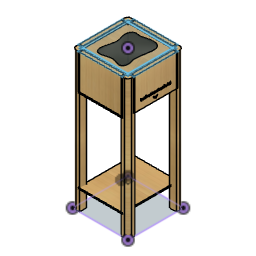
Let-me-fix-it-for-you-Final (Autodesk Fusion 360 design; units mm, degrees)
Autodesk Fusion 360 part; units mm, degrees
(part 1 of 2)
ref_plane "Plan de construction1" through (0, 1000, 0) normal (0, 1, 0) x (0, 0, 1)
sketch "Esquisse1" plane through (0, 1000, 0) normal (0, 1, 0) x (1, 0, 0)
  line L0 (200, 200) -> (-200, 200)
  line L1 (-200, 200) -> (-200, -200)
  line L2 (-200, -200) -> (200, -200)
  line L3 (200, -200) -> (200, 200)
  line L4 (200, 200) -> (-200, -200) construction
  line L5 (-200, 200) -> (200, -200) construction
  dimension "d2" = 400
  constraint horizontal L0
  constraint perpendicular L0 L1
  constraint parallel L0 L2
  constraint parallel L1 L3
  constraint coincident L4 origin
  constraint coincident L5 origin
  constraint equal L0 L1
  measures "d2" distance of L0.start L0.end
sketch "Esquisse2" plane through (0, 0, 0) normal (0, 1, 0) x (1, 0, 0)
  line L0 (200, 200) -> (-200, 200)
  line L1 (-200, 200) -> (-200, -200)
  line L2 (-200, -200) -> (200, -200)
  line L3 (200, -200) -> (200, 200)
  line L4 (-200, 200) -> (-150, 200)
  line L5 (-150, 200) -> (-150, 150)
  line L6 (-150, 150) -> (-200, 150)
  line L7 (-200, 150) -> (-200, 200)
  dimension "d3" = 50
  constraint horizontal L4
  constraint vertical L5
  constraint horizontal L6
  constraint vertical L7
  constraint coincident L0 L1.start
  constraint coincident L1 L6.end
  constraint equal L5 L6
  measures "d3" distance of L5.end L6.end
extrude "Extrusion1" add sketch "Esquisse2" along normal up to surface (1000 mm away) contours L0 L1 L4 L5 L6 L7 makes body 1
fillet "Congé1" radius 25 1 edges at (-200, 500, -200) on bodies 1
pattern_circular "Réseau C1" count 4 over 360 about axis through (0, 1.75, 0) along (0, 1, 0) of bodies 1 makes body 2 at (-150, 333.3333, 166.6667) makes body 3 at (166.6667, 333.3333, 150) makes body 4 at (150, 333.3333, -166.6667)
sketch "Esquisse6" plane through (0, 1000, 0) normal (0, 1, 0) x (1, 0, 0)
  line L0 (200, -160.0001) -> (160.0002, -160.0001)
  line L1 (160.0002, -160.0001) -> (160.0002, 160.0013)
  line L2 (160.0002, 160.0013) -> (200, 160.0013)
  line L3 (200, 160.0013) -> (200, -160.0001)
  line L4 (-160.0013, 200) -> (160.0001, 200)
  line L5 (160.0001, 160.0002) -> (-160.0013, 160.0002)
  line L6 (-160.0013, 160.0002) -> (-160.0013, 200)
  line L7 (160.0001, 200) -> (160.0001, 160.0002)
  line L8 (-200, -160.0013) -> (-200, 160.0001)
  line L9 (-160.0002, 160.0001) -> (-160.0002, -160.0013)
  line L10 (-160.0002, -160.0013) -> (-200, -160.0013)
  line L11 (-200, 160.0001) -> (-160.0002, 160.0001)
  line L12 (160.0013, -200) -> (-160.0001, -200)
  line L13 (-160.0001, -160.0002) -> (160.0013, -160.0002)
  line L14 (160.0013, -160.0002) -> (160.0013, -200)
  line L15 (-160.0001, -200) -> (-160.0001, -160.0002)
  dimension "d15" = 360
  constraint horizontal L0
  constraint vertical L1
  constraint horizontal L2
  constraint vertical L3
extrude "Extrusion2" add sketch "Esquisse6" against normal blind 230 separate body contours L0 L1 L2 L3 makes body 5
extrude "Extrusion3" add sketch "Esquisse6" against normal blind 250 separate body contours L12 L13 L14 L15 | L4 L5 L6 L7 | L8 L9 L10 L11 makes body 6 at (53.3342, 916.6667, 200) makes body 7 at (-160.0009, 916.6667, -53.333) makes body 8 at (53.333, 833.3333, -160.0009)
sketch "Esquisse15" plane through (0, 1000, 0) normal (0, 1, 0) x (1, 0, 0)
  line L0 (-175, 175) -> (175, 175)
  line L1 (175, 175) -> (175, -175)
  line L2 (175, -175) -> (-175, -175)
  line L3 (-175, -175) -> (-175, 175)
  constraint horizontal L0
  constraint vertical L1
  constraint horizontal L2
  constraint vertical L3
ref_plane "Plan de construction8" through (0, 750, 0) normal (0, 1, 0) x (1, 0, 0)
sketch "Esquisse17" plane through (0, 1000, 0) normal (0, 1, 0) x (1, 0, 0)
  line L0 (160, -200) -> (-160, -200)
  line L1 (-160, -200) -> (-160, 200)
  line L2 (-160, 200) -> (160, 200)
  line L3 (160, 200) -> (160, -200)
  constraint horizontal L0
  constraint vertical L1
  constraint horizontal L2
  constraint vertical L3
extrude "Extrusion9" add sketch "Esquisse17" against normal blind 10 from surface at -250 separate body makes body 9
extrude "Extrusion10" cut sketch "Esquisse15" against normal blind 3 bodies 1 2 3 4 5 6 7 8
extrude "Extrusion11" add sketch "Esquisse15" against normal blind 3 separate body makes body 10
ref_plane "Plan de construction9" through (0, 980, 0) normal (0, 1, 0) x (1, 0, 0)
extrude "Extrusion12" cut sketch "Esquisse15" along normal blind 3 from surface at -20 bodies 1 2 3 4 5 6 7 8
extrude "Extrusion13" add sketch "Esquisse15" along normal blind 3 from surface at -20 separate body makes body 11
sketch "Esquisse19" plane through (0, 1000, 0) normal (0, 1, 0) x (1, 0, 0)
  line L0 (107.45, 140.3) -> (-107.45, 140.3)
  line L1 (-107.45, 140.3) -> (-107.45, -140.3)
  line L2 (-107.45, -140.3) -> (107.45, -140.3)
  line L3 (107.45, -140.3) -> (107.45, 140.3)
  line L4 (107.45, 140.3) -> (-107.45, -140.3) construction
  line L5 (-107.45, 140.3) -> (107.45, -140.3) construction
  dimension "d66" = 214.9
  dimension "d67" = 280.6
  constraint horizontal L0
  constraint perpendicular L0 L1
  constraint parallel L0 L2
  constraint parallel L1 L3
  constraint coincident L4 origin
  constraint coincident L5 origin
  measures "d66" distance of L1.end L2.end
  measures "d67" distance of L0.end L1.end
extrude "Extrusion15" add sketch "Esquisse19" along normal blind 6.4 from surface at -17 bodies 11
ref_plane "Plan de construction10" through (0, 997, 0) normal (0, 1, 0) x (1, 0, 0)
extrude "Extrusion17" cut sketch "Esquisse15" against normal blind 3 from surface at -3 bodies 1 2 3 4 5 6 8 11
extrude "Extrusion18" add sketch "Esquisse15" against normal blind 3 from surface at -3 separate body makes body 12
sketch "Esquisse20" plane through (0, 1000, 0) normal (0, 1, 0) x (1, 0, 0)
  spline S0 degree 5 poles (2.9702, -120.1045) (7.0681, -119.8348) (15.2569, -119.7939) (27.4222, -121.4279) (43.0106, -127.0491) (61.2249, -134.4245) (77.5138, -136.2031) (91.0503, -127.6879) (98.8241, -110.0516) (98.8295, -90.0131) (94.6353, -72.3389) (90.1903, -60.1213) (88.8467, -53.3029) (88.4034, -45.7936) (88.4913, -33.5384) (89.8196, -15.0168) (93.0533, 9.1619) (97.7061, 35.6857) (101.4655, 59.537) (103.2857, 79.7063) (102.3989, 96.5235) (98.2065, 110.9745) (90.2444, 123.7985) (77.0958, 133.2881) (58.9031, 137.9279) (37.8289, 138.035) (16.5657, 134.6422) (-2.421, 129.4881) (-17.8557, 124.5172) (-30.8107, 121.6439) (-43.6339, 121.9352) (-58.1106, 124.5676) (-74.1441, 126.1002) (-87.4634, 118.7531) (-96.3647, 103.3877) (-100.3382, 83.9127) (-100.0369, 65.4428) (-96.4821, 49.6829) (-91.3708, 35.4015) (-86.8957, 21.1757) (-84.9832, 5.2069) (-86.8039, -13.7696) (-92.0527, -35.9447) (-98.6926, -60.0391) (-103.9624, -83.9818) (-105.043, -105.3549) (-100.0919, -121.9553) (-88.5831, -132.2499) (-73.2953, -136.0188) (-55.9982, -134.3536) (-37.333, -129.1226) (-21.5591, -124.2663) (-9.3306, -121.4124) (-1.1277, -120.3743) (2.9702, -120.1045) knots 0 0 0 0 0 0 0.02 0.04 0.06 0.08 0.1 0.12 0.14 0.16 0.18 0.2 0.22 0.24 0.26 0.28 0.3 0.32 0.34 0.36 0.38 0.4 0.42 0.44 0.46 0.48 0.5 0.52 0.54 0.56 0.58 0.6 0.62 0.64 0.66 0.68 0.7 0.72 0.74 0.76 0.78 0.8 0.82 0.84 0.86 0.88 0.9 0.92 0.94 0.96 0.98 1 1 1 1 1 1
  line L0 (-41.6235, -123.0399) -> (47.5639, -117.1691)
  line L1 (85.8055, -37.2443) -> (103.3819, 71.9806)
  line L2 (93.3383, -74.908) -> (85.8055, -37.2443)
  line L3 (71.5377, -150.9467) -> (110.117, -96.7951)
  line L4 (108.4038, 100.8562) -> (72.0487, 142.3216)
  line L5 (-102.9243, 107.4984) -> (-95.8249, 27.6746)
  line L6 (-30.9544, 124.4197) -> (-100, 125)
  line L7 (-111.5032, -112.7754) -> (-71.7545, -143.3305)
  point P0 (90.8274, -123.8709)
  point P1 (89.5719, -56.0761)
  point P2 (94.5937, 17.3682)
  point P3 (90.2262, 121.5889)
  point P4 (-5.2152, 128.4762)
  point P5 (-65.4772, 124.7099)
  point P6 (-99.3746, 67.5865)
  point P7 (-86.82, -8.9964)
  point P8 (-91.6288, -128.0529)
  constraint midpoint S0.start L0
  constraint midpoint P2 L1
  constraint midpoint P1 L2
  constraint coincident L1.start L2.end
  constraint midpoint P0 L3
  constraint midpoint P3 L4
  constraint midpoint P6 L5
  constraint midpoint P5 L6
  constraint midpoint P8 L7
extrude "Extrusion19" cut sketch "Esquisse20" against normal blind 3 from surface at -3 bodies 12
sketch "Esquisse29" plane through (200, 0, 0) normal (1, 0, 0) x (0, 0, -1)
  line L0 (-104.418, 836.9255) -> (-104.418, 820.5796)
  line L1 (-104.418, 820.5796) -> (-108.4, 820.5796)
  line L2 (-108.4, 820.5796) -> (-108.4, 836.9255)
  line L3 (-108.4, 836.9255) -> (-104.418, 836.9255)
  spline S0 degree 3 poles (-90.7629, 832.2345) (-89.8554, 831.2476) (-89.4003, 829.8956) (-89.4003, 828.1705) knots 0 0 0 0 1 1 1 1
  line L4 (-89.4003, 828.1705) -> (-89.4003, 820.5796)
  line L5 (-89.4003, 820.5796) -> (-93.3584, 820.5796)
  line L6 (-93.3584, 820.5796) -> (-93.3584, 827.6334)
  spline S1 degree 3 poles (-93.3584, 827.6334) (-93.3584, 828.5039) (-93.5833, 829.1785) (-94.0331, 829.6601) knots 0 0 0 0 1 1 1 1
  spline S2 degree 3 poles (-94.0331, 829.6601) (-94.4829, 830.1416) (-95.0888, 830.3824) (-95.8482, 830.3824) knots 0 0 0 0 1 1 1 1
  spline S3 degree 3 poles (-95.8482, 830.3824) (-96.6075, 830.3824) (-97.2134, 830.1416) (-97.6632, 829.6601) knots 0 0 0 0 1 1 1 1
  spline S4 degree 3 poles (-97.6632, 829.6601) (-98.113, 829.1785) (-98.3379, 828.5039) (-98.3379, 827.6334) knots 0 0 0 0 1 1 1 1
  line L7 (-98.3379, 827.6334) -> (-98.3379, 820.5796)
  line L8 (-98.3379, 820.5796) -> (-102.3199, 820.5796)
  line L9 (-102.3199, 820.5796) -> (-102.3199, 833.5733)
  line L10 (-102.3199, 833.5733) -> (-98.3379, 833.5733)
  line L11 (-98.3379, 833.5733) -> (-98.3379, 831.8508)
  spline S5 degree 3 poles (-98.3379, 831.8508) (-97.9357, 832.425) (-97.3907, 832.8801) (-96.7081, 833.2134) knots 0 0 0 0 1 1 1 1
  spline S6 degree 3 poles (-96.7081, 833.2134) (-96.0254, 833.5468) (-95.2581, 833.7135) (-94.4035, 833.7135) knots 0 0 0 0 1 1 1 1
  spline S7 degree 3 poles (-94.4035, 833.7135) (-92.8822, 833.7135) (-91.6677, 833.2214) (-90.7602, 832.2345) knots 0 0 0 0 1 1 1 1
  line L12 (-90.7602, 832.2345) -> (-90.7629, 832.2345)
  spline S8 degree 3 poles (-85.1643, 820.9765) (-86.048, 821.3654) (-86.7465, 821.8972) (-87.2598, 822.5719) knots 0 0 0 0 1 1 1 1
  spline S9 degree 3 poles (-87.2598, 822.5719) (-87.7731, 823.2466) (-88.0588, 824.0033) (-88.1223, 824.842) knots 0 0 0 0 1 1 1 1
  line L13 (-88.1223, 824.842) -> (-84.188, 824.842)
  spline S10 degree 3 poles (-84.188, 824.842) (-84.1404, 824.3922) (-83.9313, 824.0271) (-83.5583, 823.7466) knots 0 0 0 0 1 1 1 1
  spline S11 degree 3 poles (-83.5583, 823.7466) (-83.1852, 823.4662) (-82.7275, 823.3286) (-82.1851, 823.3286) knots 0 0 0 0 1 1 1 1
  spline S12 degree 3 poles (-82.1851, 823.3286) (-81.6877, 823.3286) (-81.304, 823.4265) (-81.0315, 823.6196) knots 0 0 0 0 1 1 1 1
  spline S13 degree 3 poles (-81.0315, 823.6196) (-80.759, 823.8128) (-80.624, 824.0668) (-80.624, 824.3764) knots 0 0 0 0 1 1 1 1
  spline S14 degree 3 poles (-80.624, 824.3764) (-80.624, 824.7494) (-80.8172, 825.0246) (-81.2061, 825.2019) knots 0 0 0 0 1 1 1 1
  spline S15 degree 3 poles (-81.2061, 825.2019) (-81.5951, 825.3791) (-82.2221, 825.5776) (-83.0926, 825.7945) knots 0 0 0 0 1 1 1 1
  spline S16 degree 3 poles (-83.0926, 825.7945) (-84.0239, 826.0115) (-84.7992, 826.2417) (-85.4209, 826.4824) knots 0 0 0 0 1 1 1 1
  spline S17 degree 3 poles (-85.4209, 826.4824) (-86.0427, 826.7232) (-86.5772, 827.1042) (-87.027, 827.6228) knots 0 0 0 0 1 1 1 1
  spline S18 degree 3 poles (-87.027, 827.6228) (-87.4767, 828.1414) (-87.7016, 828.8452) (-87.7016, 829.7289) knots 0 0 0 0 1 1 1 1
  spline S19 degree 3 poles (-87.7016, 829.7289) (-87.7016, 830.475) (-87.4953, 831.1523) (-87.0852, 831.7662) knots 0 0 0 0 1 1 1 1
  spline S20 degree 3 poles (-87.0852, 831.7662) (-86.6751, 832.38) (-86.0692, 832.8642) (-85.2701, 833.2214) knots 0 0 0 0 1 1 1 1
  spline S21 degree 3 poles (-85.2701, 833.2214) (-84.4711, 833.5786) (-83.5212, 833.7558) (-82.4179, 833.7558) knots 0 0 0 0 1 1 1 1
  spline S22 degree 3 poles (-82.4179, 833.7558) (-80.7881, 833.7558) (-79.5049, 833.351) (-78.5656, 832.544) knots 0 0 0 0 1 1 1 1
  spline S23 degree 3 poles (-78.5656, 832.544) (-77.6263, 831.7371) (-77.0866, 830.6655) (-76.9463, 829.332) knots 0 0 0 0 1 1 1 1
  line L14 (-76.9463, 829.332) -> (-80.624, 829.332)
  spline S24 degree 3 poles (-80.624, 829.332) (-80.6849, 829.7818) (-80.8833, 830.139) (-81.2167, 830.4036) knots 0 0 0 0 1 1 1 1
  spline S25 degree 3 poles (-81.2167, 830.4036) (-81.5501, 830.6681) (-81.9893, 830.8004) (-82.5317, 830.8004) knots 0 0 0 0 1 1 1 1
  spline S26 degree 3 poles (-82.5317, 830.8004) (-82.9974, 830.8004) (-83.3545, 830.7105) (-83.6032, 830.5332) knots 0 0 0 0 1 1 1 1
  spline S27 degree 3 poles (-83.6032, 830.5332) (-83.852, 830.3559) (-83.9763, 830.1099) (-83.9763, 829.8003) knots 0 0 0 0 1 1 1 1
  spline S28 degree 3 poles (-83.9763, 829.8003) (-83.9763, 829.4272) (-83.7779, 829.1494) (-83.3836, 828.9616) knots 0 0 0 0 1 1 1 1
  spline S29 degree 3 poles (-83.3836, 828.9616) (-82.9868, 828.7764) (-82.3703, 828.5885) (-81.5316, 828.4033) knots 0 0 0 0 1 1 1 1
  spline S30 degree 3 poles (-81.5316, 828.4033) (-80.5685, 828.1546) (-79.7853, 827.9112) (-79.1794, 827.6704) knots 0 0 0 0 1 1 1 1
  spline S31 degree 3 poles (-79.1794, 827.6704) (-78.5735, 827.4296) (-78.0417, 827.0407) (-77.584, 826.5062) knots 0 0 0 0 1 1 1 1
  spline S32 degree 3 poles (-77.584, 826.5062) (-77.1263, 825.9718) (-76.8908, 825.2521) (-76.8749, 824.3525) knots 0 0 0 0 1 1 1 1
  spline S33 degree 3 poles (-76.8749, 824.3525) (-76.8749, 823.5905) (-77.0892, 822.9132) (-77.5152, 822.3152) knots 0 0 0 0 1 1 1 1
  spline S34 degree 3 poles (-77.5152, 822.3152) (-77.9412, 821.7173) (-78.555, 821.249) (-79.354, 820.9077) knots 0 0 0 0 1 1 1 1
  spline S35 degree 3 poles (-79.354, 820.9077) (-80.1531, 820.5664) (-81.0818, 820.3944) (-82.1375, 820.3944) knots 0 0 0 0 1 1 1 1
  spline S36 degree 3 poles (-82.1375, 820.3944) (-83.2699, 820.3944) (-84.2806, 820.5875) (-85.1643, 820.9765) knots 0 0 0 0 1 1 1 1
  line L15 (-63.0451, 826.1226) -> (-72.0568, 826.1226)
  spline S37 degree 3 poles (-72.0568, 826.1226) (-71.996, 825.3156) (-71.734, 824.6991) (-71.2763, 824.2705) knots 0 0 0 0 1 1 1 1
  spline S38 degree 3 poles (-71.2763, 824.2705) (-70.8186, 823.8445) (-70.255, 823.6302) (-69.5883, 823.6302) knots 0 0 0 0 1 1 1 1
  spline S39 degree 3 poles (-69.5883, 823.6302) (-68.5961, 823.6302) (-67.9055, 824.0483) (-67.5166, 824.887) knots 0 0 0 0 1 1 1 1
  line L16 (-67.5166, 824.887) -> (-63.278, 824.887)
  spline S40 degree 3 poles (-63.278, 824.887) (-63.4949, 824.0324) (-63.8865, 823.2651) (-64.4527, 822.5825) knots 0 0 0 0 1 1 1 1
  spline S41 degree 3 poles (-64.4527, 822.5825) (-65.0189, 821.8999) (-65.7306, 821.3627) (-66.5826, 820.9765) knots 0 0 0 0 1 1 1 1
  spline S42 degree 3 poles (-66.5826, 820.9765) (-67.4372, 820.5875) (-68.3897, 820.3944) (-69.4454, 820.3944) knots 0 0 0 0 1 1 1 1
  spline S43 degree 3 poles (-69.4454, 820.3944) (-70.718, 820.3944) (-71.8505, 820.6669) (-72.8453, 821.2093) knots 0 0 0 0 1 1 1 1
  spline S44 degree 3 poles (-72.8453, 821.2093) (-73.8401, 821.7517) (-74.6154, 822.5296) (-75.1736, 823.5376) knots 0 0 0 0 1 1 1 1
  spline S45 degree 3 poles (-75.1736, 823.5376) (-75.7319, 824.5457) (-76.0124, 825.7257) (-76.0124, 827.0778) knots 0 0 0 0 1 1 1 1
  spline S46 degree 3 poles (-76.0124, 827.0778) (-76.0124, 828.4298) (-75.7372, 829.6072) (-75.1869, 830.6179) knots 0 0 0 0 1 1 1 1
  spline S47 degree 3 poles (-75.1869, 830.6179) (-74.6365, 831.6259) (-73.8639, 832.4038) (-72.8691, 832.9462) knots 0 0 0 0 1 1 1 1
  spline S48 degree 3 poles (-72.8691, 832.9462) (-71.8769, 833.4886) (-70.7339, 833.7611) (-69.4454, 833.7611) knots 0 0 0 0 1 1 1 1
  spline S49 degree 3 poles (-69.4454, 833.7611) (-68.1569, 833.7611) (-67.0694, 833.4965) (-66.0931, 832.97) knots 0 0 0 0 1 1 1 1
  spline S50 degree 3 poles (-66.0931, 832.97) (-65.1142, 832.4409) (-64.3522, 831.6894) (-63.7992, 830.7105) knots 0 0 0 0 1 1 1 1
  spline S51 degree 3 poles (-63.7992, 830.7105) (-63.2489, 829.7315) (-62.9737, 828.5912) (-62.9737, 827.2868) knots 0 0 0 0 1 1 1 1
  spline S52 degree 3 poles (-62.9737, 827.2868) (-62.9737, 826.9137) (-62.9975, 826.5248) (-63.0425, 826.1226) knots 0 0 0 0 1 1 1 1
  line L17 (-63.0425, 826.1226) -> (-63.0451, 826.1226)
  line L18 (-66.7705, 837.2986) -> (-66.7705, 834.5522)
  line L19 (-66.7705, 834.5522) -> (-72.3823, 836.9044)
  line L20 (-72.3823, 836.9044) -> (-72.3823, 840)
  line L21 (-72.3823, 840) -> (-66.7705, 837.2986)
  spline S53 degree 3 poles (-67.0483, 828.3345) (-67.0483, 829.0171) (-67.2811, 829.5595) (-67.7468, 829.9644) knots 0 0 0 0 1 1 1 1
  spline S54 degree 3 poles (-67.7468, 829.9644) (-68.2124, 830.3692) (-68.7945, 830.5703) (-69.493, 830.5703) knots 0 0 0 0 1 1 1 1
  spline S55 degree 3 poles (-69.493, 830.5703) (-70.1915, 830.5703) (-70.7233, 830.3771) (-71.1811, 829.9882) knots 0 0 0 0 1 1 1 1
  spline S56 degree 3 poles (-71.1811, 829.9882) (-71.6388, 829.5992) (-71.9219, 829.0489) (-72.0304, 828.3345) knots 0 0 0 0 1 1 1 1
  line L22 (-72.0304, 828.3345) -> (-67.0483, 828.3345)
  spline S57 degree 3 poles (-55.9437, 833.097) (-55.2452, 833.5071) (-54.47, 833.7135) (-53.6154, 833.7135) knots 0 0 0 0 1 1 1 1
  line L23 (-53.6154, 833.7135) -> (-53.6154, 829.4987)
  line L24 (-53.6154, 829.4987) -> (-54.7108, 829.4987)
  spline S58 degree 3 poles (-54.7108, 829.4987) (-55.7056, 829.4987) (-56.4491, 829.2844) (-56.9465, 828.8584) knots 0 0 0 0 1 1 1 1
  spline S59 degree 3 poles (-56.9465, 828.8584) (-57.4439, 828.4324) (-57.6926, 827.6836) (-57.6926, 826.6121) knots 0 0 0 0 1 1 1 1
  line L25 (-57.6926, 826.6121) -> (-57.6926, 820.5822)
  line L26 (-57.6926, 820.5822) -> (-61.6746, 820.5822)
  line L27 (-61.6746, 820.5822) -> (-61.6746, 833.5733)
  line L28 (-61.6746, 833.5733) -> (-57.6926, 833.5733)
  line L29 (-57.6926, 833.5733) -> (-57.6926, 831.409)
  spline S60 degree 3 poles (-57.6926, 831.409) (-57.2269, 832.1234) (-56.6449, 832.6869) (-55.9464, 833.097) knots 0 0 0 0 1 1 1 1
  line L30 (-55.9464, 833.097) -> (-55.9437, 833.097)
  line L31 (-40.3201, 826.1226) -> (-49.3318, 826.1226)
  spline S61 degree 3 poles (-49.3318, 826.1226) (-49.2709, 825.3156) (-49.009, 824.6991) (-48.5513, 824.2705) knots 0 0 0 0 1 1 1 1
  spline S62 degree 3 poles (-48.5513, 824.2705) (-48.0935, 823.8445) (-47.53, 823.6302) (-46.8632, 823.6302) knots 0 0 0 0 1 1 1 1
  spline S63 degree 3 poles (-46.8632, 823.6302) (-45.871, 823.6302) (-45.1805, 824.0483) (-44.7915, 824.887) knots 0 0 0 0 1 1 1 1
  line L32 (-44.7915, 824.887) -> (-40.5529, 824.887)
  spline S64 degree 3 poles (-40.5529, 824.887) (-40.7699, 824.0324) (-41.1614, 823.2651) (-41.7276, 822.5825) knots 0 0 0 0 1 1 1 1
  spline S65 degree 3 poles (-41.7276, 822.5825) (-42.2939, 821.8999) (-43.0056, 821.3627) (-43.8575, 820.9765) knots 0 0 0 0 1 1 1 1
  spline S66 degree 3 poles (-43.8575, 820.9765) (-44.7121, 820.5875) (-45.6646, 820.3944) (-46.7203, 820.3944) knots 0 0 0 0 1 1 1 1
  spline S67 degree 3 poles (-46.7203, 820.3944) (-47.993, 820.3944) (-49.1254, 820.6669) (-50.1202, 821.2093) knots 0 0 0 0 1 1 1 1
  spline S68 degree 3 poles (-50.1202, 821.2093) (-51.1151, 821.7517) (-51.8903, 822.5296) (-52.4486, 823.5376) knots 0 0 0 0 1 1 1 1
  spline S69 degree 3 poles (-52.4486, 823.5376) (-53.0068, 824.5457) (-53.2873, 825.7257) (-53.2873, 827.0778) knots 0 0 0 0 1 1 1 1
  spline S70 degree 3 poles (-53.2873, 827.0778) (-53.2873, 828.4298) (-53.0121, 829.6072) (-52.4618, 830.6179) knots 0 0 0 0 1 1 1 1
  spline S71 degree 3 poles (-52.4618, 830.6179) (-51.9115, 831.6259) (-51.1389, 832.4038) (-50.144, 832.9462) knots 0 0 0 0 1 1 1 1
  spline S72 degree 3 poles (-50.144, 832.9462) (-49.1519, 833.4886) (-48.0089, 833.7611) (-46.7203, 833.7611) knots 0 0 0 0 1 1 1 1
  spline S73 degree 3 poles (-46.7203, 833.7611) (-45.4318, 833.7611) (-44.3444, 833.4965) (-43.3681, 832.97) knots 0 0 0 0 1 1 1 1
  spline S74 degree 3 poles (-43.3681, 832.97) (-42.3891, 832.4409) (-41.6271, 831.6894) (-41.0741, 830.7105) knots 0 0 0 0 1 1 1 1
  spline S75 degree 3 poles (-41.0741, 830.7105) (-40.5238, 829.7315) (-40.2486, 828.5912) (-40.2486, 827.2868) knots 0 0 0 0 1 1 1 1
  spline S76 degree 3 poles (-40.2486, 827.2868) (-40.2486, 826.9137) (-40.2724, 826.5248) (-40.3174, 826.1226) knots 0 0 0 0 1 1 1 1
  line L33 (-40.3174, 826.1226) -> (-40.3201, 826.1226)
  spline S77 degree 3 poles (-44.3232, 828.3345) (-44.3232, 829.0171) (-44.556, 829.5595) (-45.0217, 829.9644) knots 0 0 0 0 1 1 1 1
  spline S78 degree 3 poles (-45.0217, 829.9644) (-45.4874, 830.3692) (-46.0695, 830.5703) (-46.768, 830.5703) knots 0 0 0 0 1 1 1 1
  spline S79 degree 3 poles (-46.768, 830.5703) (-47.4665, 830.5703) (-47.9983, 830.3771) (-48.456, 829.9882) knots 0 0 0 0 1 1 1 1
  spline S80 degree 3 poles (-48.456, 829.9882) (-48.9137, 829.5992) (-49.1968, 829.0489) (-49.3053, 828.3345) knots 0 0 0 0 1 1 1 1
  line L34 (-49.3053, 828.3345) -> (-44.3232, 828.3345)
  line L35 (-27.5619, 823.9583) -> (-27.5619, 820.5822)
  line L36 (-27.5619, 820.5822) -> (-29.5886, 820.5822)
  spline S81 degree 3 poles (-29.5886, 820.5822) (-31.0332, 820.5822) (-32.1577, 820.9341) (-32.9646, 821.6406) knots 0 0 0 0 1 1 1 1
  spline S82 degree 3 poles (-32.9646, 821.6406) (-33.7716, 822.347) (-34.1764, 823.5006) (-34.1764, 825.0987) knots 0 0 0 0 1 1 1 1
  line L37 (-34.1764, 825.0987) -> (-34.1764, 830.2686)
  line L38 (-34.1764, 830.2686) -> (-35.7586, 830.2686)
  line L39 (-35.7586, 830.2686) -> (-35.7586, 833.5759)
  line L40 (-35.7586, 833.5759) -> (-34.1764, 833.5759)
  line L41 (-34.1764, 833.5759) -> (-34.1764, 836.743)
  line L42 (-34.1764, 836.743) -> (-30.1945, 836.743)
  line L43 (-30.1945, 836.743) -> (-30.1945, 833.5759)
  line L44 (-30.1945, 833.5759) -> (-27.5857, 833.5759)
  line L45 (-27.5857, 833.5759) -> (-27.5857, 830.2686)
  line L46 (-27.5857, 830.2686) -> (-30.1945, 830.2686)
  line L47 (-30.1945, 830.2686) -> (-30.1945, 825.0537)
  spline S83 degree 3 poles (-30.1945, 825.0537) (-30.1945, 824.6648) (-30.1019, 824.3869) (-29.914, 824.215) knots 0 0 0 0 1 1 1 1
  spline S84 degree 3 poles (-29.914, 824.215) (-29.7288, 824.043) (-29.4166, 823.9583) (-28.9827, 823.9583) knots 0 0 0 0 1 1 1 1
  line L48 (-28.9827, 823.9583) -> (-27.5619, 823.9583)
  spline S85 degree 3 poles (-23.6619, 821.2093) (-24.6779, 821.7517) (-25.4769, 822.5296) (-26.059, 823.5376) knots 0 0 0 0 1 1 1 1
  spline S86 degree 3 poles (-26.059, 823.5376) (-26.6411, 824.5457) (-26.9321, 825.7257) (-26.9321, 827.0778) knots 0 0 0 0 1 1 1 1
  spline S87 degree 3 poles (-26.9321, 827.0778) (-26.9321, 828.4298) (-26.6385, 829.5886) (-26.0484, 830.6046) knots 0 0 0 0 1 1 1 1
  spline S88 degree 3 poles (-26.0484, 830.6046) (-25.4584, 831.6206) (-24.6514, 832.4012) (-23.6275, 832.9436) knots 0 0 0 0 1 1 1 1
  spline S89 degree 3 poles (-23.6275, 832.9436) (-22.6036, 833.486) (-21.4553, 833.7585) (-20.1826, 833.7585) knots 0 0 0 0 1 1 1 1
  spline S90 degree 3 poles (-20.1826, 833.7585) (-18.91, 833.7585) (-17.7617, 833.486) (-16.7378, 832.9436) knots 0 0 0 0 1 1 1 1
  spline S91 degree 3 poles (-16.7378, 832.9436) (-15.7138, 832.4012) (-14.9068, 831.6206) (-14.3168, 830.6046) knots 0 0 0 0 1 1 1 1
  spline S92 degree 3 poles (-14.3168, 830.6046) (-13.7268, 829.5886) (-13.4331, 828.4113) (-13.4331, 827.0778) knots 0 0 0 0 1 1 1 1
  spline S93 degree 3 poles (-13.4331, 827.0778) (-13.4331, 825.7443) (-13.7321, 824.5669) (-14.3301, 823.5509) knots 0 0 0 0 1 1 1 1
  spline S94 degree 3 poles (-14.3301, 823.5509) (-14.928, 822.5349) (-15.7429, 821.7543) (-16.7748, 821.2119) knots 0 0 0 0 1 1 1 1
  spline S95 degree 3 poles (-16.7748, 821.2119) (-17.8067, 820.6695) (-18.9603, 820.397) (-20.2329, 820.397) knots 0 0 0 0 1 1 1 1
  spline S96 degree 3 poles (-20.2329, 820.397) (-21.5056, 820.397) (-22.6512, 820.6695) (-23.6672, 821.2119) knots 0 0 0 0 1 1 1 1
  line L49 (-23.6672, 821.2119) -> (-23.6619, 821.2093)
  spline S97 degree 3 poles (-18.2829, 824.6806) (-17.7485, 825.2389) (-17.4786, 826.0379) (-17.4786, 827.0777) knots 0 0 0 0 1 1 1 1
  spline S98 degree 3 poles (-17.4786, 827.0777) (-17.4786, 828.1176) (-17.7379, 828.9166) (-18.2591, 829.4749) knots 0 0 0 0 1 1 1 1
  spline S99 degree 3 poles (-18.2591, 829.4749) (-18.7803, 830.0331) (-19.4206, 830.3136) (-20.18, 830.3136) knots 0 0 0 0 1 1 1 1
  spline S100 degree 3 poles (-20.18, 830.3136) (-20.9393, 830.3136) (-21.6008, 830.0384) (-22.1114, 829.4881) knots 0 0 0 0 1 1 1 1
  spline S101 degree 3 poles (-22.1114, 829.4881) (-22.6247, 828.9378) (-22.8787, 828.1334) (-22.8787, 827.0777) knots 0 0 0 0 1 1 1 1
  spline S102 degree 3 poles (-22.8787, 827.0777) (-22.8787, 826.0221) (-22.6274, 825.2389) (-22.122, 824.6806) knots 0 0 0 0 1 1 1 1
  spline S103 degree 3 poles (-22.122, 824.6806) (-21.6167, 824.1224) (-20.9843, 823.8419) (-20.225, 823.8419) knots 0 0 0 0 1 1 1 1
  spline S104 degree 3 poles (-20.225, 823.8419) (-19.4656, 823.8419) (-18.8174, 824.1224) (-18.2803, 824.6806) knots 0 0 0 0 1 1 1 1
  line L50 (-18.2803, 824.6806) -> (-18.2829, 824.6806)
  spline S105 degree 3 poles (-0.54, 832.2345) (0.3676, 831.2476) (0.8226, 829.8956) (0.8226, 828.1705) knots 0 0 0 0 1 1 1 1
  line L51 (0.8226, 828.1705) -> (0.8226, 820.5796)
  line L52 (0.8226, 820.5796) -> (-3.1355, 820.5796)
  line L53 (-3.1355, 820.5796) -> (-3.1355, 827.6334)
  spline S106 degree 3 poles (-3.1355, 827.6334) (-3.1355, 828.5039) (-3.3604, 829.1785) (-3.8102, 829.6601) knots 0 0 0 0 1 1 1 1
  spline S107 degree 3 poles (-3.8102, 829.6601) (-4.26, 830.1416) (-4.8659, 830.3824) (-5.6252, 830.3824) knots 0 0 0 0 1 1 1 1
  spline S108 degree 3 poles (-5.6252, 830.3824) (-6.3846, 830.3824) (-6.9905, 830.1416) (-7.4403, 829.6601) knots 0 0 0 0 1 1 1 1
  spline S109 degree 3 poles (-7.4403, 829.6601) (-7.8901, 829.1785) (-8.115, 828.5039) (-8.115, 827.6334) knots 0 0 0 0 1 1 1 1
  line L54 (-8.115, 827.6334) -> (-8.115, 820.5796)
  line L55 (-8.115, 820.5796) -> (-12.0969, 820.5796)
  line L56 (-12.0969, 820.5796) -> (-12.0969, 833.5733)
  line L57 (-12.0969, 833.5733) -> (-8.115, 833.5733)
  line L58 (-8.115, 833.5733) -> (-8.115, 831.8508)
  spline S110 degree 3 poles (-8.115, 831.8508) (-7.7128, 832.425) (-7.1678, 832.8801) (-6.4851, 833.2134) knots 0 0 0 0 1 1 1 1
  spline S111 degree 3 poles (-6.4851, 833.2134) (-5.8025, 833.5468) (-5.0352, 833.7135) (-4.1806, 833.7135) knots 0 0 0 0 1 1 1 1
  spline S112 degree 3 poles (-4.1806, 833.7135) (-2.6593, 833.7135) (-1.4448, 833.2214) (-0.5373, 832.2345) knots 0 0 0 0 1 1 1 1
  line L59 (-0.5373, 832.2345) -> (-0.54, 832.2345)
  spline S113 degree 3 poles (6.9081, 830.6179) (7.4134, 831.6259) (8.0987, 832.4038) (8.9692, 832.9462) knots 0 0 0 0 1 1 1 1
  spline S114 degree 3 poles (8.9692, 832.9462) (9.837, 833.4886) (10.808, 833.7611) (11.8796, 833.7611) knots 0 0 0 0 1 1 1 1
  spline S115 degree 3 poles (11.8796, 833.7611) (12.7342, 833.7611) (13.5121, 833.5812) (14.2185, 833.2267) knots 0 0 0 0 1 1 1 1
  spline S116 degree 3 poles (14.2185, 833.2267) (14.9249, 832.8695) (15.4806, 832.3879) (15.8827, 831.782) knots 0 0 0 0 1 1 1 1
  line L60 (15.8827, 831.782) -> (15.8827, 837.8119)
  line L61 (15.8827, 837.8119) -> (19.8647, 837.8119)
  line L62 (19.8647, 837.8119) -> (19.8647, 820.5822)
  line L63 (19.8647, 820.5822) -> (15.8827, 820.5822)
  line L64 (15.8827, 820.5822) -> (15.8827, 822.4449)
  spline S117 degree 3 poles (15.8827, 822.4449) (15.5097, 821.8231) (14.9779, 821.3284) (14.2873, 820.9553) knots 0 0 0 0 1 1 1 1
  spline S118 degree 3 poles (14.2873, 820.9553) (13.5967, 820.5822) (12.7924, 820.397) (11.8769, 820.397) knots 0 0 0 0 1 1 1 1
  spline S119 degree 3 poles (11.8769, 820.397) (10.8054, 820.397) (9.8344, 820.6722) (8.9665, 821.2225) knots 0 0 0 0 1 1 1 1
  spline S120 degree 3 poles (8.9665, 821.2225) (8.096, 821.7729) (7.4108, 822.556) (6.9054, 823.5747) knots 0 0 0 0 1 1 1 1
  spline S121 degree 3 poles (6.9054, 823.5747) (6.4001, 824.5907) (6.1487, 825.7681) (6.1487, 827.1016) knots 0 0 0 0 1 1 1 1
  spline S122 degree 3 poles (6.1487, 827.1016) (6.1487, 828.4351) (6.4001, 829.6072) (6.9054, 830.6179) knots 0 0 0 0 1 1 1 1
  line L65 (6.9054, 830.6179) -> (6.9081, 830.6179)
  spline S123 degree 3 poles (15.0572, 829.4299) (14.5069, 830.004) (13.8349, 830.2924) (13.0438, 830.2924) knots 0 0 0 0 1 1 1 1
  spline S124 degree 3 poles (13.0438, 830.2924) (12.2526, 830.2924) (11.5806, 830.0093) (11.0303, 829.4431) knots 0 0 0 0 1 1 1 1
  spline S125 degree 3 poles (11.0303, 829.4431) (10.4799, 828.8769) (10.2048, 828.0964) (10.2048, 827.1042) knots 0 0 0 0 1 1 1 1
  spline S126 degree 3 poles (10.2048, 827.1042) (10.2048, 826.112) (10.4799, 825.3236) (11.0303, 824.7415) knots 0 0 0 0 1 1 1 1
  spline S127 degree 3 poles (11.0303, 824.7415) (11.5806, 824.1594) (12.2526, 823.8684) (13.0438, 823.8684) knots 0 0 0 0 1 1 1 1
  spline S128 degree 3 poles (13.0438, 823.8684) (13.8349, 823.8684) (14.5069, 824.1541) (15.0572, 824.7309) knots 0 0 0 0 1 1 1 1
  spline S129 degree 3 poles (15.0572, 824.7309) (15.6076, 825.305) (15.8827, 826.0882) (15.8827, 827.083) knots 0 0 0 0 1 1 1 1
  spline S130 degree 3 poles (15.8827, 827.083) (15.8827, 828.0779) (15.6076, 828.861) (15.0572, 829.4352) knots 0 0 0 0 1 1 1 1
  line L66 (15.0572, 829.4352) -> (15.0572, 829.4299)
  line L67 (34.139, 826.1226) -> (25.1273, 826.1226)
  spline S131 degree 3 poles (25.1273, 826.1226) (25.1881, 825.3156) (25.4501, 824.6991) (25.9078, 824.2705) knots 0 0 0 0 1 1 1 1
  spline S132 degree 3 poles (25.9078, 824.2705) (26.3655, 823.8445) (26.9291, 823.6302) (27.5958, 823.6302) knots 0 0 0 0 1 1 1 1
  spline S133 degree 3 poles (27.5958, 823.6302) (28.588, 823.6302) (29.2812, 824.0483) (29.6675, 824.887) knots 0 0 0 0 1 1 1 1
  line L68 (29.6675, 824.887) -> (33.9062, 824.887)
  spline S134 degree 3 poles (33.9062, 824.887) (33.6892, 824.0324) (33.2976, 823.2651) (32.7314, 822.5825) knots 0 0 0 0 1 1 1 1
  spline S135 degree 3 poles (32.7314, 822.5825) (32.1652, 821.8999) (31.4535, 821.3627) (30.6015, 820.9765) knots 0 0 0 0 1 1 1 1
  spline S136 degree 3 poles (30.6015, 820.9765) (29.7469, 820.5875) (28.7944, 820.3944) (27.7387, 820.3944) knots 0 0 0 0 1 1 1 1
  spline S137 degree 3 poles (27.7387, 820.3944) (26.4661, 820.3944) (25.3337, 820.6669) (24.3388, 821.2093) knots 0 0 0 0 1 1 1 1
  spline S138 degree 3 poles (24.3388, 821.2093) (23.3466, 821.7517) (22.5688, 822.5296) (22.0105, 823.5376) knots 0 0 0 0 1 1 1 1
  spline S139 degree 3 poles (22.0105, 823.5376) (21.4522, 824.5457) (21.1718, 825.7257) (21.1718, 827.0778) knots 0 0 0 0 1 1 1 1
  spline S140 degree 3 poles (21.1718, 827.0778) (21.1718, 828.4298) (21.4469, 829.6072) (21.9973, 830.6179) knots 0 0 0 0 1 1 1 1
  spline S141 degree 3 poles (21.9973, 830.6179) (22.5476, 831.6259) (23.3202, 832.4038) (24.315, 832.9462) knots 0 0 0 0 1 1 1 1
  spline S142 degree 3 poles (24.315, 832.9462) (25.3072, 833.4886) (26.4502, 833.7611) (27.7387, 833.7611) knots 0 0 0 0 1 1 1 1
  spline S143 degree 3 poles (27.7387, 833.7611) (29.0272, 833.7611) (30.1147, 833.4965) (31.091, 832.97) knots 0 0 0 0 1 1 1 1
  spline S144 degree 3 poles (31.091, 832.97) (32.0699, 832.4409) (32.8319, 831.6894) (33.3849, 830.7105) knots 0 0 0 0 1 1 1 1
  spline S145 degree 3 poles (33.3849, 830.7105) (33.9353, 829.7315) (34.2104, 828.5912) (34.2104, 827.2868) knots 0 0 0 0 1 1 1 1
  spline S146 degree 3 poles (34.2104, 827.2868) (34.2104, 826.9137) (34.1866, 826.5248) (34.1416, 826.1226) knots 0 0 0 0 1 1 1 1
  line L69 (34.1416, 826.1226) -> (34.139, 826.1226)
  spline S147 degree 3 poles (30.1332, 828.3345) (30.1332, 829.0171) (29.9004, 829.5595) (29.4347, 829.9644) knots 0 0 0 0 1 1 1 1
  spline S148 degree 3 poles (29.4347, 829.9644) (28.969, 830.3692) (28.3869, 830.5703) (27.6884, 830.5703) knots 0 0 0 0 1 1 1 1
  spline S149 degree 3 poles (27.6884, 830.5703) (26.99, 830.5703) (26.4581, 830.3771) (26.0004, 829.9882) knots 0 0 0 0 1 1 1 1
  spline S150 degree 3 poles (26.0004, 829.9882) (25.5427, 829.5992) (25.2596, 829.0489) (25.1511, 828.3345) knots 0 0 0 0 1 1 1 1
  line L70 (25.1511, 828.3345) -> (30.1332, 828.3345)
  spline S151 degree 3 poles (37.7717, 820.9765) (36.888, 821.3654) (36.1895, 821.8972) (35.6762, 822.5719) knots 0 0 0 0 1 1 1 1
  spline S152 degree 3 poles (35.6762, 822.5719) (35.1629, 823.2466) (34.8772, 824.0033) (34.8137, 824.842) knots 0 0 0 0 1 1 1 1
  line L71 (34.8137, 824.842) -> (38.748, 824.842)
  spline S153 degree 3 poles (38.748, 824.842) (38.7957, 824.3922) (39.0047, 824.0271) (39.3777, 823.7466) knots 0 0 0 0 1 1 1 1
  spline S154 degree 3 poles (39.3777, 823.7466) (39.7508, 823.4662) (40.2085, 823.3286) (40.7509, 823.3286) knots 0 0 0 0 1 1 1 1
  spline S155 degree 3 poles (40.7509, 823.3286) (41.2483, 823.3286) (41.632, 823.4265) (41.9045, 823.6196) knots 0 0 0 0 1 1 1 1
  spline S156 degree 3 poles (41.9045, 823.6196) (42.177, 823.8128) (42.312, 824.0668) (42.312, 824.3764) knots 0 0 0 0 1 1 1 1
  spline S157 degree 3 poles (42.312, 824.3764) (42.312, 824.7494) (42.1188, 825.0246) (41.7299, 825.2019) knots 0 0 0 0 1 1 1 1
  spline S158 degree 3 poles (41.7299, 825.2019) (41.3409, 825.3791) (40.7139, 825.5776) (39.8434, 825.7945) knots 0 0 0 0 1 1 1 1
  spline S159 degree 3 poles (39.8434, 825.7945) (38.9121, 826.0115) (38.1368, 826.2417) (37.5151, 826.4824) knots 0 0 0 0 1 1 1 1
  spline S160 degree 3 poles (37.5151, 826.4824) (36.8933, 826.7232) (36.3588, 827.1042) (35.909, 827.6228) knots 0 0 0 0 1 1 1 1
  spline S161 degree 3 poles (35.909, 827.6228) (35.4592, 828.1414) (35.2344, 828.8452) (35.2344, 829.7289) knots 0 0 0 0 1 1 1 1
  spline S162 degree 3 poles (35.2344, 829.7289) (35.2344, 830.475) (35.4407, 831.1523) (35.8508, 831.7662) knots 0 0 0 0 1 1 1 1
  spline S163 degree 3 poles (35.8508, 831.7662) (36.2609, 832.38) (36.8668, 832.8642) (37.6659, 833.2214) knots 0 0 0 0 1 1 1 1
  spline S164 degree 3 poles (37.6659, 833.2214) (38.4649, 833.5786) (39.4148, 833.7558) (40.5181, 833.7558) knots 0 0 0 0 1 1 1 1
  spline S165 degree 3 poles (40.5181, 833.7558) (42.1479, 833.7558) (43.4312, 833.351) (44.3704, 832.544) knots 0 0 0 0 1 1 1 1
  spline S166 degree 3 poles (44.3704, 832.544) (45.3097, 831.7371) (45.8495, 830.6655) (45.9897, 829.332) knots 0 0 0 0 1 1 1 1
  line L72 (45.9897, 829.332) -> (42.312, 829.332)
  spline S167 degree 3 poles (42.312, 829.332) (42.2485, 829.7818) (42.0527, 830.139) (41.7193, 830.4036) knots 0 0 0 0 1 1 1 1
  spline S168 degree 3 poles (41.7193, 830.4036) (41.3859, 830.6681) (40.9467, 830.8004) (40.4043, 830.8004) knots 0 0 0 0 1 1 1 1
  spline S169 degree 3 poles (40.4043, 830.8004) (39.9387, 830.8004) (39.5815, 830.7105) (39.3328, 830.5332) knots 0 0 0 0 1 1 1 1
  spline S170 degree 3 poles (39.3328, 830.5332) (39.0841, 830.3559) (38.9597, 830.1099) (38.9597, 829.8003) knots 0 0 0 0 1 1 1 1
  spline S171 degree 3 poles (38.9597, 829.8003) (38.9597, 829.4272) (39.1581, 829.1494) (39.5524, 828.9616) knots 0 0 0 0 1 1 1 1
  spline S172 degree 3 poles (39.5524, 828.9616) (39.9492, 828.7764) (40.5657, 828.5885) (41.4045, 828.4033) knots 0 0 0 0 1 1 1 1
  spline S173 degree 3 poles (41.4045, 828.4033) (42.3675, 828.1546) (43.1507, 827.9112) (43.7566, 827.6704) knots 0 0 0 0 1 1 1 1
  spline S174 degree 3 poles (43.7566, 827.6704) (44.3625, 827.4296) (44.8943, 827.0407) (45.352, 826.5062) knots 0 0 0 0 1 1 1 1
  spline S175 degree 3 poles (45.352, 826.5062) (45.8098, 825.9718) (46.0453, 825.2521) (46.0611, 824.3525) knots 0 0 0 0 1 1 1 1
  spline S176 degree 3 poles (46.0611, 824.3525) (46.0611, 823.5905) (45.8468, 822.9132) (45.4208, 822.3152) knots 0 0 0 0 1 1 1 1
  spline S177 degree 3 poles (45.4208, 822.3152) (44.9949, 821.7173) (44.381, 821.249) (43.582, 820.9077) knots 0 0 0 0 1 1 1 1
  spline S178 degree 3 poles (43.582, 820.9077) (42.7829, 820.5664) (41.8542, 820.3944) (40.7986, 820.3944) knots 0 0 0 0 1 1 1 1
  spline S179 degree 3 poles (40.7986, 820.3944) (39.6661, 820.3944) (38.6554, 820.5875) (37.7717, 820.9765) knots 0 0 0 0 1 1 1 1
  spline S180 degree 3 poles (49.9716, 820.9765) (49.0879, 821.3654) (48.3894, 821.8972) (47.8762, 822.5719) knots 0 0 0 0 1 1 1 1
  spline S181 degree 3 poles (47.8762, 822.5719) (47.3629, 823.2466) (47.0771, 824.0033) (47.0136, 824.842) knots 0 0 0 0 1 1 1 1
  line L73 (47.0136, 824.842) -> (50.948, 824.842)
  spline S182 degree 3 poles (50.948, 824.842) (50.9956, 824.3922) (51.2046, 824.0271) (51.5777, 823.7466) knots 0 0 0 0 1 1 1 1
  spline S183 degree 3 poles (51.5777, 823.7466) (51.9507, 823.4662) (52.4085, 823.3286) (52.9509, 823.3286) knots 0 0 0 0 1 1 1 1
  spline S184 degree 3 poles (52.9509, 823.3286) (53.4483, 823.3286) (53.8319, 823.4265) (54.1044, 823.6196) knots 0 0 0 0 1 1 1 1
  spline S185 degree 3 poles (54.1044, 823.6196) (54.377, 823.8128) (54.5119, 824.0668) (54.5119, 824.3764) knots 0 0 0 0 1 1 1 1
  spline S186 degree 3 poles (54.5119, 824.3764) (54.5119, 824.7494) (54.3187, 825.0246) (53.9298, 825.2019) knots 0 0 0 0 1 1 1 1
  spline S187 degree 3 poles (53.9298, 825.2019) (53.5409, 825.3791) (52.9138, 825.5776) (52.0433, 825.7945) knots 0 0 0 0 1 1 1 1
  spline S188 degree 3 poles (52.0433, 825.7945) (51.112, 826.0115) (50.3368, 826.2417) (49.715, 826.4824) knots 0 0 0 0 1 1 1 1
  spline S189 degree 3 poles (49.715, 826.4824) (49.0932, 826.7232) (48.5588, 827.1042) (48.109, 827.6228) knots 0 0 0 0 1 1 1 1
  spline S190 degree 3 poles (48.109, 827.6228) (47.6592, 828.1414) (47.4343, 828.8452) (47.4343, 829.7289) knots 0 0 0 0 1 1 1 1
  spline S191 degree 3 poles (47.4343, 829.7289) (47.4343, 830.475) (47.6407, 831.1523) (48.0508, 831.7662) knots 0 0 0 0 1 1 1 1
  spline S192 degree 3 poles (48.0508, 831.7662) (48.4609, 832.38) (49.0668, 832.8642) (49.8658, 833.2214) knots 0 0 0 0 1 1 1 1
  spline S193 degree 3 poles (49.8658, 833.2214) (50.6649, 833.5786) (51.6147, 833.7558) (52.718, 833.7558) knots 0 0 0 0 1 1 1 1
  spline S194 degree 3 poles (52.718, 833.7558) (54.3479, 833.7558) (55.6311, 833.351) (56.5704, 832.544) knots 0 0 0 0 1 1 1 1
  spline S195 degree 3 poles (56.5704, 832.544) (57.5096, 831.7371) (58.0494, 830.6655) (58.1896, 829.332) knots 0 0 0 0 1 1 1 1
  line L74 (58.1896, 829.332) -> (54.5119, 829.332)
  spline S196 degree 3 poles (54.5119, 829.332) (54.4484, 829.7818) (54.2526, 830.139) (53.9192, 830.4036) knots 0 0 0 0 1 1 1 1
  spline S197 degree 3 poles (53.9192, 830.4036) (53.5858, 830.6681) (53.1466, 830.8004) (52.6043, 830.8004) knots 0 0 0 0 1 1 1 1
  spline S198 degree 3 poles (52.6043, 830.8004) (52.1386, 830.8004) (51.7814, 830.7105) (51.5327, 830.5332) knots 0 0 0 0 1 1 1 1
  spline S199 degree 3 poles (51.5327, 830.5332) (51.284, 830.3559) (51.1596, 830.1099) (51.1596, 829.8003) knots 0 0 0 0 1 1 1 1
  spline S200 degree 3 poles (51.1596, 829.8003) (51.1596, 829.4272) (51.3581, 829.1494) (51.7523, 828.9616) knots 0 0 0 0 1 1 1 1
  spline S201 degree 3 poles (51.7523, 828.9616) (52.1492, 828.7764) (52.7657, 828.5885) (53.6044, 828.4033) knots 0 0 0 0 1 1 1 1
  spline S202 degree 3 poles (53.6044, 828.4033) (54.5675, 828.1546) (55.3506, 827.9112) (55.9565, 827.6704) knots 0 0 0 0 1 1 1 1
  spline S203 degree 3 poles (55.9565, 827.6704) (56.5624, 827.4296) (57.0942, 827.0407) (57.552, 826.5062) knots 0 0 0 0 1 1 1 1
  spline S204 degree 3 poles (57.552, 826.5062) (58.0097, 825.9718) (58.2452, 825.2521) (58.2611, 824.3525) knots 0 0 0 0 1 1 1 1
  spline S205 degree 3 poles (58.2611, 824.3525) (58.2611, 823.5905) (58.0468, 822.9132) (57.6208, 822.3152) knots 0 0 0 0 1 1 1 1
  spline S206 degree 3 poles (57.6208, 822.3152) (57.1948, 821.7173) (56.581, 821.249) (55.7819, 820.9077) knots 0 0 0 0 1 1 1 1
  spline S207 degree 3 poles (55.7819, 820.9077) (54.9829, 820.5664) (54.0542, 820.3944) (52.9985, 820.3944) knots 0 0 0 0 1 1 1 1
  spline S208 degree 3 poles (52.9985, 820.3944) (51.8661, 820.3944) (50.8554, 820.5875) (49.9716, 820.9765) knots 0 0 0 0 1 1 1 1
  spline S209 degree 3 poles (60.2031, 835.5418) (59.7612, 835.9519) (59.539, 836.4625) (59.539, 837.0658) knots 0 0 0 0 1 1 1 1
  spline S210 degree 3 poles (59.539, 837.0658) (59.539, 837.669) (59.7612, 838.2035) (60.2031, 838.6136) knots 0 0 0 0 1 1 1 1
  spline S211 degree 3 poles (60.2031, 838.6136) (60.6449, 839.0237) (61.2164, 839.2301) (61.9149, 839.2301) knots 0 0 0 0 1 1 1 1
  spline S212 degree 3 poles (61.9149, 839.2301) (62.6134, 839.2301) (63.1611, 839.0237) (63.603, 838.6136) knots 0 0 0 0 1 1 1 1
  spline S213 degree 3 poles (63.603, 838.6136) (64.0448, 838.2035) (64.2671, 837.6849) (64.2671, 837.0658) knots 0 0 0 0 1 1 1 1
  spline S214 degree 3 poles (64.2671, 837.0658) (64.2671, 836.4466) (64.0448, 835.9519) (63.603, 835.5418) knots 0 0 0 0 1 1 1 1
  spline S215 degree 3 poles (63.603, 835.5418) (63.1611, 835.1317) (62.5976, 834.9253) (61.9149, 834.9253) knots 0 0 0 0 1 1 1 1
  spline S216 degree 3 poles (61.9149, 834.9253) (61.2323, 834.9253) (60.6449, 835.1317) (60.2031, 835.5418) knots 0 0 0 0 1 1 1 1
  line L75 (63.894, 833.5733) -> (63.894, 820.5822)
  line L76 (63.894, 820.5822) -> (59.912, 820.5822)
  line L77 (59.912, 820.5822) -> (59.912, 833.5733)
  line L78 (59.912, 833.5733) -> (63.894, 833.5733)
  spline S217 degree 3 poles (77.5518, 832.2345) (78.4593, 831.2476) (78.9144, 829.8956) (78.9144, 828.1705) knots 0 0 0 0 1 1 1 1
  line L79 (78.9144, 828.1705) -> (78.9144, 820.5796)
  line L80 (78.9144, 820.5796) -> (74.9562, 820.5796)
  line L81 (74.9563, 820.5796) -> (74.9563, 827.6334)
  spline S218 degree 3 poles (74.9563, 827.6334) (74.9563, 828.5039) (74.7314, 829.1785) (74.2816, 829.6601) knots 0 0 0 0 1 1 1 1
  spline S219 degree 3 poles (74.2816, 829.6601) (73.8318, 830.1416) (73.2259, 830.3824) (72.4665, 830.3824) knots 0 0 0 0 1 1 1 1
  spline S220 degree 3 poles (72.4665, 830.3824) (71.7072, 830.3824) (71.1013, 830.1416) (70.6515, 829.6601) knots 0 0 0 0 1 1 1 1
  spline S221 degree 3 poles (70.6515, 829.6601) (70.2017, 829.1785) (69.9768, 828.5039) (69.9768, 827.6334) knots 0 0 0 0 1 1 1 1
  line L82 (69.9768, 827.6334) -> (69.9768, 820.5796)
  line L83 (69.9768, 820.5796) -> (65.9948, 820.5796)
  line L84 (65.9948, 820.5796) -> (65.9948, 833.5733)
  line L85 (65.9948, 833.5733) -> (69.9768, 833.5733)
  line L86 (69.9768, 833.5733) -> (69.9768, 831.8508)
  spline S222 degree 3 poles (69.9768, 831.8508) (70.3816, 832.425) (70.924, 832.8801) (71.6066, 833.2134) knots 0 0 0 0 1 1 1 1
  spline S223 degree 3 poles (71.6066, 833.2134) (72.2893, 833.5468) (73.0565, 833.7135) (73.9112, 833.7135) knots 0 0 0 0 1 1 1 1
  spline S224 degree 3 poles (73.9112, 833.7135) (75.4325, 833.7135) (76.647, 833.2214) (77.5545, 832.2345) knots 0 0 0 0 1 1 1 1
  line L87 (77.5545, 832.2345) -> (77.5518, 832.2345)
  spline S225 degree 3 poles (85.3253, 835.5418) (84.8834, 835.9519) (84.6612, 836.4625) (84.6612, 837.0658) knots 0 0 0 0 1 1 1 1
  spline S226 degree 3 poles (84.6612, 837.0658) (84.6612, 837.669) (84.8834, 838.2035) (85.3253, 838.6136) knots 0 0 0 0 1 1 1 1
  spline S227 degree 3 poles (85.3253, 838.6136) (85.7671, 839.0237) (86.3386, 839.2301) (87.0371, 839.2301) knots 0 0 0 0 1 1 1 1
  spline S228 degree 3 poles (87.0371, 839.2301) (87.7356, 839.2301) (88.2833, 839.0237) (88.7252, 838.6136) knots 0 0 0 0 1 1 1 1
  spline S229 degree 3 poles (88.7252, 838.6136) (89.167, 838.2035) (89.3893, 837.6849) (89.3893, 837.0658) knots 0 0 0 0 1 1 1 1
  spline S230 degree 3 poles (89.3893, 837.0658) (89.3893, 836.4466) (89.167, 835.9519) (88.7252, 835.5418) knots 0 0 0 0 1 1 1 1
  spline S231 degree 3 poles (88.7252, 835.5418) (88.2833, 835.1317) (87.7197, 834.9253) (87.0371, 834.9253) knots 0 0 0 0 1 1 1 1
  spline S232 degree 3 poles (87.0371, 834.9253) (86.3545, 834.9253) (85.7671, 835.1317) (85.3253, 835.5418) knots 0 0 0 0 1 1 1 1
  line L88 (89.0162, 833.5733) -> (89.0162, 820.5822)
  line L89 (89.0162, 820.5822) -> (85.0342, 820.5822)
  line L90 (85.0342, 820.5822) -> (85.0342, 833.5733)
  line L91 (85.0342, 833.5733) -> (89.0162, 833.5733)
  spline S233 degree 3 poles (91.1488, 830.6179) (91.6991, 831.6259) (92.469, 832.4038) (93.4533, 832.9462) knots 0 0 0 0 1 1 1 1
  spline S234 degree 3 poles (93.4533, 832.9462) (94.4375, 833.4886) (95.5673, 833.7611) (96.8399, 833.7611) knots 0 0 0 0 1 1 1 1
  spline S235 degree 3 poles (96.8399, 833.7611) (98.4698, 833.7611) (99.8324, 833.3351) (100.9251, 832.4805) knots 0 0 0 0 1 1 1 1
  spline S236 degree 3 poles (100.9251, 832.4805) (102.0178, 831.6259) (102.7375, 830.4247) (103.0788, 828.8716) knots 0 0 0 0 1 1 1 1
  line L92 (103.0788, 828.8716) -> (98.8402, 828.8716)
  spline S237 degree 3 poles (98.8402, 828.8716) (98.483, 829.8638) (97.7924, 830.3612) (96.7685, 830.3612) knots 0 0 0 0 1 1 1 1
  spline S238 degree 3 poles (96.7685, 830.3612) (96.0382, 830.3612) (95.4562, 830.0781) (95.0223, 829.5119) knots 0 0 0 0 1 1 1 1
  spline S239 degree 3 poles (95.0223, 829.5119) (94.5883, 828.9457) (94.3714, 828.1334) (94.3714, 827.0777) knots 0 0 0 0 1 1 1 1
  spline S240 degree 3 poles (94.3714, 827.0777) (94.3714, 826.0221) (94.5883, 825.2124) (95.0223, 824.6436) knots 0 0 0 0 1 1 1 1
  spline S241 degree 3 poles (95.0223, 824.6436) (95.4562, 824.0774) (96.0383, 823.7943) (96.7685, 823.7943) knots 0 0 0 0 1 1 1 1
  spline S242 degree 3 poles (96.7685, 823.7943) (97.7924, 823.7943) (98.483, 824.2917) (98.8402, 825.2839) knots 0 0 0 0 1 1 1 1
  line L93 (98.8402, 825.2839) -> (103.0788, 825.2839)
  spline S243 degree 3 poles (103.0788, 825.2839) (102.7375, 823.7625) (102.0152, 822.5666) (100.9145, 821.6988) knots 0 0 0 0 1 1 1 1
  spline S244 degree 3 poles (100.9145, 821.6988) (99.8112, 820.8283) (98.4539, 820.3944) (96.8399, 820.3944) knots 0 0 0 0 1 1 1 1
  spline S245 degree 3 poles (96.8399, 820.3944) (95.5673, 820.3944) (94.4375, 820.6669) (93.4533, 821.2093) knots 0 0 0 0 1 1 1 1
  spline S246 degree 3 poles (93.4533, 821.2093) (92.4664, 821.7517) (91.6991, 822.5296) (91.1488, 823.5376) knots 0 0 0 0 1 1 1 1
  spline S247 degree 3 poles (91.1488, 823.5376) (90.5984, 824.5457) (90.3233, 825.7257) (90.3233, 827.0778) knots 0 0 0 0 1 1 1 1
  spline S248 degree 3 poles (90.3233, 827.0778) (90.3233, 828.4298) (90.5984, 829.6072) (91.1488, 830.6179) knots 0 0 0 0 1 1 1 1
  spline S249 degree 3 poles (104.6981, 835.5418) (104.2562, 835.9519) (104.0339, 836.4625) (104.0339, 837.0658) knots 0 0 0 0 1 1 1 1
  spline S250 degree 3 poles (104.0339, 837.0658) (104.0339, 837.669) (104.2562, 838.2035) (104.6981, 838.6136) knots 0 0 0 0 1 1 1 1
  spline S251 degree 3 poles (104.6981, 838.6136) (105.1399, 839.0237) (105.7114, 839.2301) (106.4099, 839.2301) knots 0 0 0 0 1 1 1 1
  spline S252 degree 3 poles (106.4099, 839.2301) (107.1084, 839.2301) (107.6561, 839.0237) (108.0979, 838.6136) knots 0 0 0 0 1 1 1 1
  spline S253 degree 3 poles (108.0979, 838.6136) (108.5398, 838.2035) (108.7621, 837.6849) (108.7621, 837.0658) knots 0 0 0 0 1 1 1 1
  spline S254 degree 3 poles (108.7621, 837.0658) (108.7621, 836.4466) (108.5398, 835.9519) (108.0979, 835.5418) knots 0 0 0 0 1 1 1 1
  spline S255 degree 3 poles (108.0979, 835.5418) (107.6561, 835.1317) (107.0925, 834.9253) (106.4099, 834.9253) knots 0 0 0 0 1 1 1 1
  spline S256 degree 3 poles (106.4099, 834.9253) (105.7273, 834.9253) (105.1399, 835.1317) (104.6981, 835.5418) knots 0 0 0 0 1 1 1 1
  line L94 (108.389, 833.5733) -> (108.389, 820.5822)
  line L95 (108.389, 820.5822) -> (104.407, 820.5822)
  line L96 (104.407, 820.5822) -> (104.407, 833.5733)
  line L97 (104.407, 833.5733) -> (108.389, 833.5733)
  spline S257 degree 3 poles (17.1951, 805.4692) (16.8829, 805.2496) (0.2194, 793.2031) (0.1189, 793.1264) knots 0 0 0 0 1 1 1 1
  line L98 (0.1189, 793.1264) -> (-0.0082, 793.0285)
  line L99 (-0.0082, 793.0285) -> (-8.5198, 799.1827)
  spline S258 degree 3 poles (-8.5198, 799.1827) (-13.2003, 802.5667) (-17.0817, 805.3766) (-17.1479, 805.4269) knots 0 0 0 0 1 1 1 1
  line L100 (-17.1479, 805.4269) -> (-17.2696, 805.5195)
  line L101 (-17.2696, 805.5195) -> (-17.2696, 794.9229)
  line L102 (-17.2696, 794.9229) -> (-8.6415, 788.6841)
  line L103 (-8.6415, 788.6841) -> (-0.0134, 782.4425)
  line L104 (-0.0134, 782.4425) -> (0.1771, 782.5801)
  spline S259 degree 3 poles (0.1771, 782.5801) (0.2803, 782.6569) (4.1643, 785.4641) (8.8104, 788.8243) knots 0 0 0 0 1 1 1 1
  line L105 (8.8104, 788.8243) -> (17.2586, 794.9335)
  line L106 (17.2586, 794.9335) -> (17.2586, 805.5195)
  line L107 (17.2586, 805.5195) -> (17.1951, 805.5195)